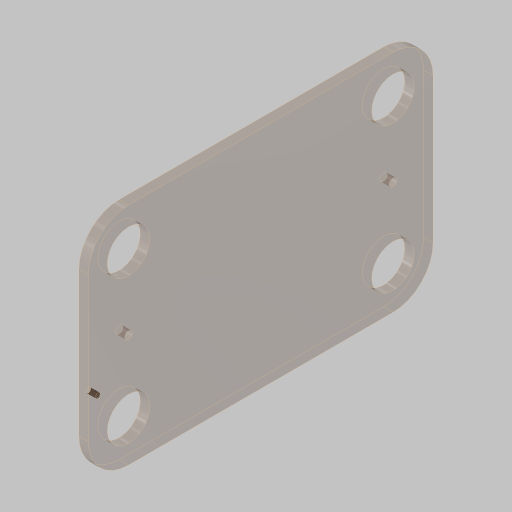
# Autodesk Inventor part: GP4-006
Saved by Autodesk Inventor 2023.5 (Build 275446000, 446)
## iProperties
Created: 2025-01-30
Part Number: GP4-006
Material: Polycarbonate, Smoke
Document SubType Name: Sheet Metal
Designer: slick
Density: 1.2 g/cm^3
Appearance: Polycarbonate - Smoked
Sheet Metal Rule: Default_mm
Author: slick
Autodesk Inventor part; units mm, degrees
ref_plane "YZ Plane" through (0, 0, 0) normal (1, 0, 0) x (0, 1, 0)
ref_plane "XZ Plane" through (0, 0, 0) normal (0, 1, 0) x (-1, 0, 0)
ref_plane "XY Plane" through (0, 0, 0) normal (0, 0, 1) x (1, 0, 0)
sketch "Sketch1" plane through (0, 0, 0) normal (1, 0, 0) x (0, 1, 0)
  circle A0 centre (0, 0) radius 14.2875
  circle A1 centre (0, -177.8) radius 14.2875
  line L0 (152.4, -31.75) -> (-152.4, -31.75) construction
  line L1 (-152.4, -31.75) -> (-152.4, -146.05) construction
  line L2 (-152.4, -146.05) -> (152.4, -146.05) construction
  line L3 (152.4, -146.05) -> (152.4, -31.75) construction
  line L4 (152.4, -31.75) -> (-152.4, -146.05) construction
  line L5 (-152.4, -31.75) -> (152.4, -146.05) construction
  circle A2 centre (0, 0) radius 38.1 construction
  circle A3 centre (0, -177.8) radius 38.1 construction
  circle A4 centre (0, 0) radius 31.75 construction
  circle A5 centre (0, -177.8) radius 31.75 construction
  circle A6 centre (0, 0) radius 26.9875 construction
  circle A7 centre (0, -177.8) radius 26.9875 construction
  circle A8 centre (97.4242, -177.8) radius 14.2875
  circle A9 centre (97.4242, -177.8) radius 38.1 construction
  circle A10 centre (97.4242, -177.8) radius 31.75 construction
  circle A11 centre (97.4242, -177.8) radius 26.9875 construction
  circle A12 centre (97.4242, 0) radius 14.2875
  circle A13 centre (97.4242, 0) radius 38.1 construction
  circle A14 centre (97.4242, 0) radius 31.75 construction
  circle A15 centre (97.4242, 0) radius 26.9875 construction
  line L6 (97.4242, -204.7875) -> (0, -204.7875)
  line L7 (97.4242, 26.9875) -> (0, 26.9875)
  line L8 (124.4117, 0) -> (124.4117, -177.8)
  line L9 (-26.9875, 0) -> (-26.9875, -177.8)
  arc A16 (124.4117, 0) -> (97.4242, 26.9875) centre (97.4242, 0) ccw
  arc A17 (97.4242, -204.7875) -> (124.4117, -177.8) centre (97.4242, -177.8) ccw
  arc A18 (0, 26.9875) -> (-26.9875, 0) centre (0, 0) ccw
  arc A19 (-26.9875, -177.8) -> (0, -204.7875) centre (0, -177.8) ccw
  line L10 (97.4242, -177.8) -> (0, -177.8) construction
  point P0 (0, -88.9)
  point P1 (48.7121, 0)
  point P2 (48.7121, -177.8)
  point P3 (48.7121, -177.8)
  dimension "d0" = 28.575
  dimension "d2" = 304.8
  dimension "d3" = 114.3
  dimension "d4" = 76.2
  dimension "d6" = 6.35
  dimension "d7" = 12.7
  dimension "d8" = 97.4242
  constraints: 22 end point, 20 centre point, 18 point on circle, 16 coincident, 13 equal radius, 9 tangent, 4 horizontal alignment, 4 vertical alignment, 3 midpoint, 3 parallel, 2 horizontal, 1 perpendicular
  measures "d0" diameter of A0
  measures "d2" distance of L2.end L1.end
  measures "d3" distance of L1.end L0.end
  measures "d4" diameter of A2
  measures "d6" radial gap between concentric circles of A2 A4
  measures "d7" radial gap between concentric circles of A0 A6
  measures "d8" distance of point (0, 0) A12.centre
extrude "Extrusion1" add sketch "Sketch1" along normal blind 6.35
hole "Hole1" at (0, 48.7121, 0) at (0, 48.7121, -177.8) direction (1, 0, 0) diameter 5.1054 end through all clearance for "Flat Head Machine Screw (82)" size "#10" standard "Ansi Unified Screw Threads"
sketch "Sketch3" plane through (6.35, 0, 0) normal (1, 0, 0) x (0, 0, -1)
  line L0 (-26.9875, 97.4242) -> (-26.9875, 0) construction
  line L1 (0, -26.9875) -> (177.8, -26.9875) construction
  point P0 (0, 0)
  point P1 (-20.6375, 23.8125)
  dimension "d29" = 6.35
  dimension "d30" = 50.8
  measures "d29" distance from line of point (-20.637, 23.812) L0
  measures "d30" distance from line of L1 point (-20.637, 23.812)
hole "Hole2" at (6.35, 23.8125, 20.6375) direction (-1, 0, 0) diameter 3.302 end through all thread size "8-32 UNC" class "2B" standard "ANSI Unified Screw Threads"
equation "\"d36\" = Thickness"
equation "\"BendRadius\" = Thickness"
equation "\"BendReliefWidth\" = Thickness"
equation "\"BendReliefDepth\" = 0.5 * Thickness"
equation "\"CornerReliefSize\" = 4 * Thickness"
equation "\"MinimumRemnant\" = 2 * Thickness"
equation "\"TransitionRadius\" = BendRadius"
equation "\"JacobiRadiusSize\" = BendRadius"
equation "\"GapSize\" = Thickness"
equation "\"d18\" = Thickness"
equation "\"Thickness\" = 6.35"
body "Solid1"
